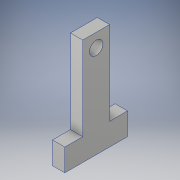
# Autodesk Inventor part: Roller Mount
Saved by Autodesk Inventor 2019.4 (Build 234330000, 330)
## iProperties
Created: 2020-01-11
Part Number: Roller Mount
Material: Aluminum 6061
Document SubType Name: Modeling
Designer: admin
Density: 2.7 g/cm^3
Appearance: Aluminum - Flat
Author: admin
Autodesk Inventor part; units mm, degrees
ref_plane "YZ Plane" through (0, 0, 0) normal (1, 0, 0) x (0, 1, 0)
ref_plane "XZ Plane" through (0, 0, 0) normal (0, 1, 0) x (-1, 0, 0)
ref_plane "XY Plane" through (0, 0, 0) normal (0, 0, 1) x (1, 0, 0)
sketch "Sketch2" plane through (0, 0, 0) normal (1, 0, 0) x (0, 1, 0)
  line L0 (0, 0) -> (0, -28)
  line L1 (0, -28) -> (10, -28)
  line L2 (10, -28) -> (10, -20)
  line L3 (10, -20) -> (47.4, -20)
  line L4 (47.4, -20) -> (47.4, -8)
  line L5 (47.4, -8) -> (10, -8)
  line L6 (10, -8) -> (10, 0)
  line L7 (10, 0) -> (0, 0)
  circle A0 centre (41.4, -14) radius 3
  line L8 (41.4, -14) -> (47.4, -14) construction
  dimension "d12" = 8
  dimension "d13" = 8
  dimension "d14" = 12
  dimension "d15" = 6
  dimension "d16" = 6
  dimension "d17" = 6
  dimension "d18" = 41.4
  dimension "d19" = 10
  constraints: 18 end point, 6 perpendicular, 2 point on line, 1 centre point, 1 midpoint, 1 vertical
  measures "d12" distance of L1.end L2.end
  measures "d13" distance of L5.end L6.end
  measures "d14" distance of L3.end L4.end
  measures "d15" diameter of A0
  measures "d16" distance of L8.start L8.end
  measures "d17" distance from line of L3 L8.start
  measures "d18" distance from line of L0 L8.start
  measures "d19" distance of L0.end L1.end
extrude "Extrusion2" add sketch "Sketch2" along normal blind 5.5
equation "\"d16\" = 0.5 * d14"
equation "\"d17\" = d16"
body "Solid2"
